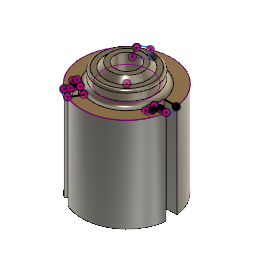
Loeffel-mitte (Autodesk Fusion 360 design; units mm, degrees)
Autodesk Fusion 360 part; units mm, degrees
note: some values were not read from the file. Set by a fixed rule: which sketch regions a step uses.
sketch "Skizze1" plane through (0, 0, 0) normal (0, 0, 1) x (1, 0, 0)
  circle A0 centre (0, 0) radius 9.5
  dimension "d1" = 19
  measures "d1" diameter of A0
extrude "Extrusion1" add sketch "Skizze1" along normal blind 20
sketch "Skizze2" plane through (0, 0, 20) normal (0, 0, 1) x (-1, 0, 0)
  circle A0 centre (0, 0) radius 9.5
  circle A1 centre (0, 0) radius 5
  dimension "d4" = 10
  measures "d4" diameter of A1
extrude "Extrusion2" add sketch "Skizze2" along normal blind 4 contours A1 picked at (1.310136, -1.993515)
sketch "Skizze3" plane through (0, 0, 24) normal (0, 0, 1) x (-1, 0, 0)
  circle A0 centre (0, 0) radius 5
  circle A1 centre (0, 0) radius 2.5
  dimension "d7" = 5
  measures "d7" diameter of A1
extrude "Extrusion3" cut sketch "Skizze3" against normal blind 38 contours A1 picked at (-0.886301, 0.232065)
sketch "Skizze4" plane through (0, 0, 20) normal (0, 0, 1) x (-1, 0, 0)
  circle A0 centre (0, 0) radius 9.5
  line L0 (-10, -1) -> (-6.928203, -1)
  line L1 (-6.911738, 1.108094) -> (-6.911738, 2.1)
  line L2 (-6.911738, 2.1) -> (-7.6, 2.1)
  line L3 (-7.6, 2.1) -> (-8.1, 1.1)
  line L4 (-8.1, 1.1) -> (-10, 1.1)
  line L5 (-10, 1.1) -> (-10, -1)
  line L6 (-6.928203, -1) -> (-6.911738, 1.108094)
  line L7 (3.097372, -7.564806) -> (4.047372, -9.210254)
  line L8 (1.981347, -7.631793) -> (3.097372, -7.564806)
  line L9 (1.637216, -7.035741) -> (1.981347, -7.631793)
  line L10 (2.496232, -6.539788) -> (1.637216, -7.035741)
  line L11 (4.330127, -5.5) -> (2.496232, -6.539788)
  line L12 (5.866025, -8.160254) -> (4.330127, -5.5)
  line L13 (4.047372, -9.210254) -> (5.866025, -8.160254)
  line L14 (5.002628, 6.464806) -> (5.952628, 8.110254)
  line L15 (5.618653, 5.531793) -> (5.002628, 6.464806)
  line L16 (5.274523, 4.935741) -> (5.618653, 5.531793)
  line L17 (4.415507, 5.431694) -> (5.274523, 4.935741)
  line L18 (2.598076, 6.5) -> (4.415507, 5.431694)
  line L19 (4.133975, 9.160254) -> (2.598076, 6.5)
  line L20 (5.952628, 8.110254) -> (4.133975, 9.160254)
  circle A1 centre (0, 0) radius 5
  dimension "d14" = 360
extrude "Extrusion4" cut sketch "Skizze4" against normal blind 23 contours A0 L14 L15 L16 L17 L18 L19 | A0 L7 L8 L9 L10 L11 L12 | A0 L0 L1 L2 L3 L4 L6 picked at (4.029402, 7.112705) picked at (4.145082, -7.045917) picked at (-8.174485, -0.066788)
sketch "Skizze5" plane through (0, 0, 0) normal (0, 0, -1) x (1, 0, 0)
  circle A0 centre (0, 0) radius 2.5
  line L0 (-3.857585, 8.681534) -> (-2.598076, 6.5)
  line L1 (-4.415507, 5.431694) -> (-5.274523, 4.935741)
  line L2 (-5.274523, 4.935741) -> (-5.618653, 5.531793)
  line L3 (-5.618653, 5.531793) -> (-5.002628, 6.464806)
  line L4 (-5.002628, 6.464806) -> (-5.670678, 7.621903)
  line L5 (-5.589636, -7.681534) -> (-4.330127, -5.5)
  line L6 (-2.496232, -6.539788) -> (-1.637216, -7.035741)
  line L7 (-1.637216, -7.035741) -> (-1.981347, -7.631793)
  line L8 (-1.981347, -7.631793) -> (-3.097372, -7.564806)
  line L9 (-3.097372, -7.564806) -> (-3.765423, -8.721903)
  line L10 (9.447222, -1) -> (6.928203, -1)
  line L11 (6.911738, 1.108094) -> (6.911738, 2.1)
  line L12 (6.911738, 2.1) -> (7.6, 2.1)
  line L13 (7.6, 2.1) -> (8.1, 1.1)
  line L14 (8.1, 1.1) -> (9.436101, 1.1)
  line L15 (4.365453, -2.43779) -> (4.293915, 2.561698)
  line L16 (4.293915, 2.561698) -> (-0.071538, 4.999488)
  line L17 (-0.071538, 4.999488) -> (-4.365453, 2.43779)
  line L18 (-4.365453, 2.43779) -> (-4.293915, -2.561698)
  line L19 (-4.293915, -2.561698) -> (0.071538, -4.999488)
  line L20 (0.071538, -4.999488) -> (4.365453, -2.43779)
  circle A1 centre (0, 0) radius 5
  circle A2 centre (0, 0) radius 5
  line L21 (-2.598076, 6.5) -> (-4.415507, 5.431694)
  line L22 (-4.330127, -5.5) -> (-2.496232, -6.539788)
  line L23 (6.928203, -1) -> (6.911738, 1.108094)
  line L24 (4, 2.309401) -> (0, 4.618802)
  line L25 (0, 4.618802) -> (-4, 2.309401)
  line L26 (-4, 2.309401) -> (-4, -2.309401)
  line L27 (-4, -2.309401) -> (0, -4.618802)
  line L28 (0, -4.618802) -> (4, -2.309401)
  line L29 (4, -2.309401) -> (4, 2.309401)
  arc A3 (-5.670678, 7.621903) -> (-5.589636, -7.681534) centre (0, 0) ccw
  arc A4 (-3.765423, -8.721903) -> (9.447222, -1) centre (0, 0) ccw
  arc A5 (9.436101, 1.1) -> (-3.857585, 8.681534) centre (0, 0) ccw
  dimension "d48" = 4.365453
  dimension "d49" = 4
  measures "d49" distance of A0.centre L29
extrude "Extrusion12" cut sketch "Skizze5" against normal blind 8 contours L24 L25 L26 L27 L28 L29 picked at (-1.75, -3.031089)
chamfer "Fase4" distance 1.5 angle 45 1 edges at (2.330818, -0.904039, 8)
chamfer "Fase5" distance 1 angle 45 1 edges at (4.661637, 1.808077, 24)
sketch "Skizze6" plane through (0, 0, 20) normal (0, 0, 1) x (-1, 0, 0)
  line L0 (-6.928203, -1) -> (-9.447222, -1)
  arc A0 (3.857585, 8.681534) -> (-9.436101, 1.1) centre (0, 0) ccw
  line L1 (3.765423, -8.721903) -> (3.097372, -7.564806)
  line L2 (3.097372, -7.564806) -> (1.981347, -7.631793)
  line L3 (1.981347, -7.631793) -> (1.637216, -7.035741)
  line L4 (1.637216, -7.035741) -> (2.496232, -6.539788)
  line L5 (-7.6, 2.1) -> (-8, 2.1)
  line L6 (-8, 2.1) -> (-8.5, 1.1)
  line L7 (-8.5, 1.1) -> (-8.1, 1.1)
  line L8 (-8.1, 1.1) -> (-7.6, 2.1)
  line L9 (2.181347, -7.978203) -> (3.297372, -7.911216)
  line L10 (3.297372, -7.911216) -> (3.097372, -7.564806)
  line L11 (3.097372, -7.564806) -> (1.981347, -7.631793)
  line L12 (1.981347, -7.631793) -> (2.181347, -7.978203)
  line L13 (5.818653, 5.878203) -> (5.202628, 6.811216)
  line L14 (5.202628, 6.811216) -> (5.002628, 6.464806)
  line L15 (5.002628, 6.464806) -> (5.618653, 5.531793)
  line L16 (5.618653, 5.531793) -> (5.818653, 5.878203)
  line L17 (2.598076, 6.5) -> (3.857585, 8.681534)
  line L18 (-9.436101, 1.1) -> (-8.1, 1.1)
  line L19 (-8.1, 1.1) -> (-7.6, 2.1)
  line L20 (-7.6, 2.1) -> (-6.911738, 2.1)
  line L21 (-6.911738, 2.1) -> (-6.911738, 1.108094)
  line L22 (-6.911738, 1.108094) -> (-6.928203, -1)
  line L23 (2.496232, -6.539788) -> (4.330127, -5.5)
  line L24 (4.330127, -5.5) -> (5.589636, -7.681534)
  arc A1 (5.589636, -7.681534) -> (5.670678, 7.621903) centre (0, 0) ccw
  line L25 (5.670678, 7.621903) -> (5.002628, 6.464806)
  line L26 (5.002628, 6.464806) -> (5.618653, 5.531793)
  line L27 (5.618653, 5.531793) -> (5.274523, 4.935741)
  line L28 (5.274523, 4.935741) -> (4.415507, 5.431694)
  line L29 (4.415507, 5.431694) -> (2.598076, 6.5)
  circle A2 centre (0, 0) radius 5
  arc A3 (-9.447222, -1) -> (3.765423, -8.721903) centre (0, 0) ccw
  dimension "d22" = 360
extrude "Extrusion6" cut sketch "Skizze6" against normal blind 22 contours L1 L2 L9 L10 L11 L12 | L5 L6 L7 L8 L18 L19 | L13 L14 L15 L16 L25 L26 picked at (2.420022, -7.724934) picked at (-8.2, 1.433333) picked at (5.479978, 5.958267)
sketch "Skizze7" plane through (0, 0, 20) normal (0, 0, 1) x (1, 0, 0)
sketch "Skizze8" plane through (0, 0, 20) normal (0, 0, 1) x (-1, 0, 0)
sketch "Skizze9" plane through (0, 0, 20) normal (0, 0, 1) x (-1, 0, 0)
  line L0 (-8.5, 1.1) -> (-8, 2.1)
  line L1 (-8, 2.1) -> (-6.911738, 2.1)
  line L2 (-6.911738, 2.1) -> (-6.911738, 1.108094)
  line L3 (2.598076, 6.5) -> (3.857585, 8.681534)
  arc A0 (5.589636, -7.681534) -> (5.670678, 7.621903) centre (0, 0) ccw
  line L4 (-9.436101, 1.1) -> (-8.5, 1.1)
  line L5 (-6.911738, 2.1) -> (-6.911738, 2.9)
  line L6 (-6.911738, 2.9) -> (-7.6, 2.9)
  line L7 (-7.6, 2.9) -> (-8, 2.1)
  line L8 (-8, 2.1) -> (-6.911738, 2.1)
  line L9 (2.181347, -7.978203) -> (1.637216, -7.035741)
  line L10 (1.288526, -8.031793) -> (2.181347, -7.978203)
  line L11 (0.944396, -7.435741) -> (1.288526, -8.031793)
  line L12 (1.637216, -7.035741) -> (0.944396, -7.435741)
  line L13 (5.818653, 5.878203) -> (5.274523, 4.935741)
  line L14 (6.311474, 5.131793) -> (5.818653, 5.878203)
  line L15 (5.967343, 4.535741) -> (6.311474, 5.131793)
  line L16 (5.274523, 4.935741) -> (5.967343, 4.535741)
  circle A1 centre (0, 0) radius 5
  line L17 (3.297372, -7.911216) -> (2.181347, -7.978203)
  line L18 (2.181347, -7.978203) -> (1.637216, -7.035741)
  line L19 (1.637216, -7.035741) -> (2.496232, -6.539788)
  line L20 (2.496232, -6.539788) -> (4.330127, -5.5)
  line L21 (4.330127, -5.5) -> (5.589636, -7.681534)
  line L22 (5.670678, 7.621903) -> (5.202628, 6.811216)
  line L23 (5.202628, 6.811216) -> (5.818653, 5.878203)
  line L24 (5.818653, 5.878203) -> (5.274523, 4.935741)
  line L25 (5.274523, 4.935741) -> (4.415507, 5.431694)
  line L26 (4.415507, 5.431694) -> (2.598076, 6.5)
  line L27 (-6.911738, 1.108094) -> (-6.928203, -1)
  line L28 (-6.928203, -1) -> (-9.447222, -1)
  arc A2 (-9.447222, -1) -> (3.765423, -8.721903) centre (0, 0) ccw
  line L29 (3.765423, -8.721903) -> (3.297372, -7.911216)
  arc A3 (3.857585, 8.681534) -> (-9.436101, 1.1) centre (0, 0) ccw
  dimension "d26" = 360
extrude "Extrusion7" cut sketch "Skizze9" against normal blind 23 contours L1 L5 L6 L7 L8 | L13 L14 L15 L16 L24 | L9 L10 L11 L12 L18 picked at (-7.503913, 2.366667) picked at (5.80155, 5.315246) picked at (1.702363, -7.681912)
sketch "Skizze10" plane through (0, 0, 20) normal (0, 0, 1) x (-1, 0, 0)
  line L0 (3.297372, -7.911216) -> (1.288526, -8.031793)
  line L1 (1.288526, -8.031793) -> (0.944396, -7.435741)
  line L2 (0.944396, -7.435741) -> (2.496232, -6.539788)
  line L3 (-6.928203, -1) -> (-9.447222, -1)
  arc A0 (-9.447222, -1) -> (3.765423, -8.721903) centre (0, 0) ccw
  line L4 (3.765423, -8.721903) -> (3.297372, -7.911216)
  line L5 (-9.447222, -1) -> (-6.895372, -1)
  line L6 (-6.895372, -1) -> (-6.895372, -1.2)
  line L7 (-6.895372, -1.2) -> (-9.447222, -1.2)
  line L8 (-9.447222, -1.2) -> (-9.447222, -1)
  line L9 (4.486917, -5.371568) -> (5.762841, -7.581534)
  line L10 (5.589636, -7.681534) -> (4.313712, -5.471568)
  line L11 (5.762841, -7.581534) -> (5.589636, -7.681534)
  line L12 (4.313712, -5.471568) -> (4.486917, -5.371568)
  line L13 (2.408456, 6.571568) -> (3.68438, 8.781534)
  line L14 (3.857585, 8.681534) -> (2.581661, 6.471568)
  line L15 (3.68438, 8.781534) -> (3.857585, 8.681534)
  line L16 (2.581661, 6.471568) -> (2.408456, 6.571568)
  line L17 (-8.5, 1.1) -> (-7.6, 2.9)
  line L18 (-7.6, 2.9) -> (-6.911738, 2.9)
  line L19 (-6.911738, 2.9) -> (-6.911738, 1.108094)
  line L20 (-6.911738, 1.108094) -> (-6.928203, -1)
  line L21 (2.496232, -6.539788) -> (4.330127, -5.5)
  line L22 (4.330127, -5.5) -> (5.589636, -7.681534)
  arc A1 (5.589636, -7.681534) -> (5.670678, 7.621903) centre (0, 0) ccw
  line L23 (5.670678, 7.621903) -> (5.202628, 6.811216)
  line L24 (5.202628, 6.811216) -> (6.311474, 5.131793)
  line L25 (6.311474, 5.131793) -> (5.967343, 4.535741)
  line L26 (5.967343, 4.535741) -> (4.415507, 5.431694)
  line L27 (4.415507, 5.431694) -> (2.598076, 6.5)
  line L28 (2.598076, 6.5) -> (3.857585, 8.681534)
  arc A2 (3.857585, 8.681534) -> (-9.436101, 1.1) centre (0, 0) ccw
  line L29 (-9.436101, 1.1) -> (-8.5, 1.1)
  circle A3 centre (0, 0) radius 5
  dimension "d29" = 0.2
  dimension "d31" = 360
extrude "Extrusion8" cut sketch "Skizze10" against normal blind 23 contours L3 A0 L5 L6 L7 | L9 L10 L12 L22 A1 | L9 L11 A1 | L13 L14 L16 L28 A2 | L13 L15 A2 picked at (-7.74916, -1.133333) picked at (4.856076, -6.144303) picked at (5.737214, -7.581554) picked at (2.893085, 7.277636) picked at (3.697211, 8.75935)
sketch "Skizze11" plane through (0, 0, 0) normal (0, 0, -1) x (1, 0, 0)
  line L0 (-4.313712, -5.471568) -> (-4.330127, -5.5)
  line L1 (-2.496232, -6.539788) -> (-0.944396, -7.435741)
  line L2 (-0.944396, -7.435741) -> (-1.288526, -8.031793)
  line L3 (-1.288526, -8.031793) -> (-3.297372, -7.911216)
  line L4 (9.423906, -1.2) -> (6.895372, -1.2)
  line L5 (6.911738, 1.108094) -> (6.911738, 2.9)
  line L6 (6.911738, 2.9) -> (7.6, 2.9)
  line L7 (7.6, 2.9) -> (8.5, 1.1)
  line L8 (-3.672722, 8.761342) -> (-2.408456, 6.571568)
  line L9 (-2.408456, 6.571568) -> (-2.581661, 6.471568)
  line L10 (-2.581661, 6.471568) -> (-2.598076, 6.5)
  line L11 (-4.415507, 5.431694) -> (-5.967343, 4.535741)
  line L12 (-5.967343, 4.535741) -> (-6.311474, 5.131793)
  line L13 (-6.311474, 5.131793) -> (-5.202628, 6.811216)
  line L14 (-5.751183, -7.561342) -> (-4.486917, -5.371568)
  line L15 (-4.486917, -5.371568) -> (-4.313712, -5.471568)
  line L16 (7.1, 2.9) -> (6.7, 2.9)
  line L17 (6.7, 2.9) -> (6.7, -1.2)
  line L18 (6.7, -1.2) -> (7.1, -1.2)
  line L19 (7.1, -1.2) -> (7.1, 2.9)
  line L20 (-5.861474, 4.35237) -> (-2.310769, 6.40237)
  line L21 (-2.510769, 6.74878) -> (-6.061474, 4.69878)
  line L22 (-2.310769, 6.40237) -> (-2.510769, 6.74878)
  line L23 (-6.061474, 4.69878) -> (-5.861474, 4.35237)
  line L24 (-0.838526, -7.25237) -> (-4.38923, -5.20237)
  line L25 (-4.58923, -5.54878) -> (-1.038526, -7.59878)
  line L26 (-4.38923, -5.20237) -> (-4.58923, -5.54878)
  line L27 (-1.038526, -7.59878) -> (-0.838526, -7.25237)
  line L28 (-4.330127, -5.5) -> (-2.496232, -6.539788)
  line L29 (6.895372, -1.2) -> (6.895372, -1)
  line L30 (6.895372, -1) -> (6.928203, -1)
  line L31 (6.928203, -1) -> (6.911738, 1.108094)
  line L32 (-2.598076, 6.5) -> (-4.415507, 5.431694)
  line L33 (0, 4.618802) -> (4, 2.309401)
  line L34 (4, 2.309401) -> (4, -2.309401)
  line L35 (4, -2.309401) -> (0, -4.618802)
  line L36 (0, -4.618802) -> (-4, -2.309401)
  line L37 (-4, -2.309401) -> (-4, 2.309401)
  line L38 (-4, 2.309401) -> (0, 4.618802)
  line L39 (-3.297372, -7.911216) -> (-3.765423, -8.721903)
  arc A0 (-3.765423, -8.721903) -> (9.423906, -1.2) centre (0, 0) ccw
  line L40 (8.5, 1.1) -> (9.436101, 1.1)
  arc A1 (9.436101, 1.1) -> (-3.672722, 8.761342) centre (0, 0) ccw
  line L41 (-5.202628, 6.811216) -> (-5.670678, 7.621903)
  arc A2 (-5.670678, 7.621903) -> (-5.751183, -7.561342) centre (0, 0) ccw
  dimension "d35" = 360
extrude "Extrusion9" cut sketch "Skizze11" against normal blind 21 contours L0 L1 L15 L24 L26 L27 L28 | L9 L10 L11 L20 L22 L23 L32 | L5 L16 L17 L18 L29 L30 L31 picked at (-2.574663, -6.331509) picked at (-4.195917, 5.395478) picked at (6.770579, 0.936031)
chamfer "Fase2" [no effect]
delete_face "Fläche löschen1" [no effect]
sketch "Skizze12" plane through (0, 0, 20) normal (0, 0, 1) x (-1, 0, 0)
  line L0 (6.311474, 5.131793) -> (5.861474, 4.35237)
  line L1 (5.861474, 4.35237) -> (2.310769, 6.40237)
  line L2 (2.310769, 6.40237) -> (3.672722, 8.761342)
  arc A0 (3.672722, 8.761342) -> (-9.436101, 1.1) centre (0, 0) ccw
  line L3 (-9.436101, 1.1) -> (-8.5, 1.1)
  line L4 (-8.5, 1.1) -> (-7.6, 2.9)
  line L5 (-7.6, 2.9) -> (-6.7, 2.9)
  line L6 (-6.7, 2.9) -> (-6.7, -1.2)
  line L7 (-6.7, -1.2) -> (-9.423906, -1.2)
  arc A1 (-9.423906, -1.2) -> (3.765423, -8.721903) centre (0, 0) ccw
  line L8 (3.765423, -8.721903) -> (3.297372, -7.911216)
  line L9 (3.297372, -7.911216) -> (1.288526, -8.031793)
  line L10 (1.288526, -8.031793) -> (0.838526, -7.25237)
  line L11 (0.838526, -7.25237) -> (4.38923, -5.20237)
  line L12 (4.38923, -5.20237) -> (5.751183, -7.561342)
  arc A2 (5.751183, -7.561342) -> (5.670678, 7.621903) centre (0, 0) ccw
  line L13 (5.670678, 7.621903) -> (5.202628, 6.811216)
  line L14 (5.202628, 6.811216) -> (6.311474, 5.131793)
  circle A3 centre (0, 0) radius 5
  circle A4 centre (0, 0) radius 6
  dimension "d39" = 12
  measures "d39" diameter of A4
extrude "Extrusion10" add sketch "Skizze12" along normal blind 4 contours A4 picked at (5.625713, -0.546488)
sketch "Skizze13" plane through (0, 0, 24) normal (0, 0, 1) x (-1, 0, 0)
  circle A0 centre (0, 0) radius 6
  circle A1 centre (0, 0) radius 2.5
  circle A2 centre (0, 0) radius 3.5
  circle A3 centre (0, 0) radius 4
  circle A4 centre (0, 0) radius 5
  dimension "d42" = 7
  measures "d42" diameter of A2
extrude "Extrusion11" cut sketch "Skizze13" against normal blind 1 contours A0 | A3 | A4 picked at (5.625713, -0.546488) picked at (3.818441, -0.198723) picked at (4.633159, -0.447127)
chamfer "Fase3" distance 1 angle 45 1 edges at (3.263146, 1.265654, 23)
fillet "Abrundung4" radius 0.5 1 edges at (5.593964, -2.169693, 23)
fillet "Abrundung5" radius 1 1 edges at (5.593964, -2.169693, 20)
